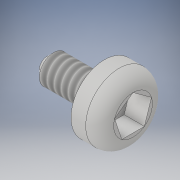
# Autodesk Inventor part: hex nut
Saved by Autodesk Inventor 2017.1 (Build 211199000, 199)
## iProperties
Created: 2017-04-27
Part Number: hex nut
Material: Generic
Document SubType Name: Modeling
Designer: 196918
Density: 1 g/cm^3
Appearance: Default
Author: 196918
Autodesk Inventor part; units mm, degrees
ref_plane "YZ Plane" through (0, 0, 0) normal (1, 0, 0) x (0, 1, 0)
ref_plane "XZ Plane" through (0, 0, 0) normal (0, 1, 0) x (-1, 0, 0)
ref_plane "XY Plane" through (0, 0, 0) normal (0, 0, 1) x (1, 0, 0)
sketch "Sketch1" plane through (0, 0, 0) normal (1, 0, 0) x (0, 1, 0)
  circle A0 centre (0, 0) radius 1.6256
  dimension "d0" = 3.2512
  constraints: 1 centre point, 1 coincident
  measures "d0" diameter of A0
extrude "Extrusion1" add sketch "Sketch1" along normal blind 3.2512
thread "Thread1" size "6-32 UNC" class "2A" standard "ANSI Unified Screw Threads" full length
sketch "Sketch2" plane through (3.2512, 0, 0) normal (1, 0, 0) x (0, 0, -1)
  circle A0 centre (0, 0) radius 1.6256
  constraints: 1 centre point, 1 coincident
extrude "Extrusion2" add sketch "Sketch2" along normal blind 3.2512
sketch "Sketch3" plane through (6.5024, 0, 0) normal (1, 0, 0) x (0, 0, -1)
  circle A0 centre (0, 0) radius 3.7786
  constraints: 1 centre point, 1 coincident
extrude "Extrusion3" add sketch "Sketch3" along normal blind 3.2512
fillet "Fillet1" radius 1.5875 1 edges at (9.7536, 0, 3.7786)
sketch "Sketch4" plane through (9.7536, 0, 0) normal (1, 0, 0) x (0, 0, -1)
  circle A0 centre (0, 0) radius 2.1911 projected
  line L0 (0, 2.1911) -> (2.0838, 0.6771)
  line L1 (2.0838, 0.6771) -> (1.2879, -1.7726)
  line L2 (1.2879, -1.7726) -> (-1.2879, -1.7726)
  line L3 (-1.2879, -1.7726) -> (-2.0838, 0.6771)
  line L4 (-2.0838, 0.6771) -> (0, 2.1911)
  constraints: 10 end point, 1 coincident, 1 vertical alignment, 12 other
extrude "Extrusion4" cut sketch "Sketch4" against normal blind 2.2987 contours L1 L2 L3 L4 L0
chamfer "Chamfer1" distance 0.762 angle 45 1 edges at (0, -1.6256, 0)
body "Solid1"
